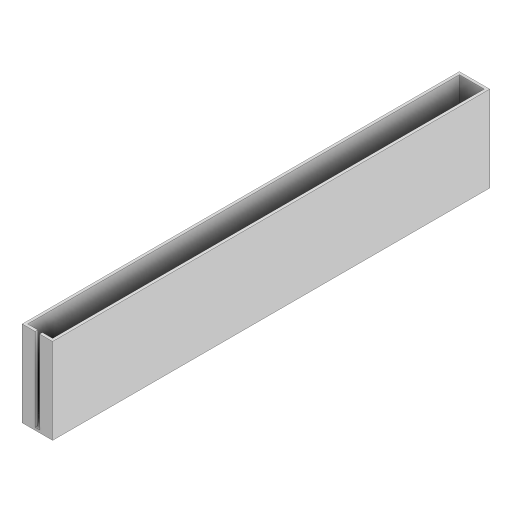
# Autodesk Inventor part: Wall Lift Test Case
Saved by Autodesk Inventor 2024.2 (Build 282272000, 272)
## iProperties
Created: 2024-12-02
Part Number: Wall Lift Test Case
Material: Generic
Document SubType Name: Modeling
Designer: rhond
Density: 1 g/cm^3
Appearance: Default
Author: rhond
Autodesk Inventor part; units mm, degrees
ref_plane "YZ Plane" through (0, 0, 0) normal (1, 0, 0) x (0, 1, 0)
ref_plane "XZ Plane" through (0, 0, 0) normal (0, 1, 0) x (-1, 0, 0)
ref_plane "XY Plane" through (0, 0, 0) normal (0, 0, 1) x (1, 0, 0)
sketch "Sketch1" plane through (0, 0, 0) normal (0, 1, 0) x (-1, 0, 0)
  line L0 (0, 0) -> (17.9705, 0)
  line L1 (17.9705, 0) -> (17.9705, -259.2705)
  line L2 (17.9705, -259.2705) -> (0, -259.2705)
  line L3 (0, -259.2705) -> (0, 0)
  dimension "d0" = 17.9705
  dimension "d1" = 259.2705
  constraints: 8 end point, 2 parallel, 1 horizontal, 1 perpendicular
  measures "d0" distance of L1.end L2.end
  measures "d1" distance of L0.end L1.end
extrude "Extrusion1" add sketch "Sketch1" along normal blind 50.8
shell "Shell1" thickness 1.5875 removed faces 1 at (-5.9902, 50.8, -172.847)
sketch "Sketch2" plane through (-17.9705, 0, 0) normal (0, 0, 1) x (1, 0, 0)
  line L0 (17.9705, 50.8) -> (0, 50.8) projected
  line L1 (1.5875, 1.5875) -> (16.383, 1.5875) projected
  line L2 (1.5875, 50.8) -> (16.383, 50.8)
  line L3 (16.383, 50.8) -> (16.383, 1.5875)
  line L4 (16.383, 1.5875) -> (1.5875, 1.5875)
  line L5 (1.5875, 1.5875) -> (1.5875, 50.8)
  line L6 (1.5875, 1.5875) -> (1.5875, 50.8) projected
  line L7 (7.6835, 50.8) -> (7.6835, 1.5875)
  line L8 (10.287, 50.8) -> (10.287, 1.5875)
  point P0 (17.9705, 0)
  point P1 (10.287, 1.5875)
  point P2 (7.6835, 1.5875)
  dimension "d5" = 0
  dimension "d6" = 6.096
  dimension "d7" = 6.096
  constraints: 12 end point, 5 point on line, 3 perpendicular, 2 parallel, 1 horizontal
  measures "d5" distance between parallel lines of L6 L5
  measures "d6" distance between parallel lines of L5 L7
  measures "d7" distance between parallel lines of L3 L8
extrude "Extrusion2" cut sketch "Sketch2" against normal blind 1.5875 contours L8 L1 L7 L0
body "Solid1"
